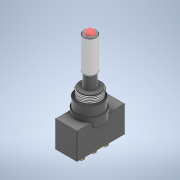
# Autodesk Inventor part: Тумблер(укороченный)
Saved by Autodesk Inventor 2020 (Build 240168000, 168)
## iProperties
Created: 2020-02-08
Part Number: Тумблер(укороченный)
Material: Типовые
Document SubType Name: Modeling
Designer: Andre
Density: 1 g/cm^3
Appearance: По умолчанию
Author: Andre
Autodesk Inventor part; units mm, degrees
ref_plane "YZ Plane" through (0, 0, 0) normal (1, 0, 0) x (0, 1, 0)
ref_plane "XZ Plane" through (0, 0, 0) normal (0, 1, 0) x (-1, 0, 0)
ref_plane "XY Plane" through (0, 0, 0) normal (0, 0, 1) x (1, 0, 0)
sketch "Эскиз1" plane through (0, 0, 0) normal (0, 1, 0) x (-1, 0, 0)
  line L0 (6, -13.1) -> (-6, -13.1)
  line L1 (-6, -13.1) -> (-6, 13.1)
  line L2 (-6, 13.1) -> (6, 13.1)
  line L3 (6, 13.1) -> (6, -13.1)
  point P0 (0, 0)
  point P1 (0, 0)
  point P2 (0, 0)
  point P3 (0, 0)
  point P4 (-5.9706, -15.2069)
  dimension "d0" = 12
  dimension "d1" = 26.2
  constraints: 8 end point, 3 coincident, 2 parallel, 1 horizontal, 1 perpendicular
  measures "d0" distance of L1.end L2.end
  measures "d1" distance of L0.end L1.end
extrude "Корпус" add sketch "Эскиз1" along normal blind 14.5
sketch "Эскиз2" plane through (0, 0, 0) normal (0, -1, 0) x (1, 0, 0)
  line L0 (3.2, 0.4) -> (-3.2, 0.4)
  line L1 (-3.2, 0.4) -> (-3.2, -0.4)
  line L2 (-3.2, -0.4) -> (3.2, -0.4)
  line L3 (3.2, -0.4) -> (3.2, 0.4)
  line L4 (3.2, -6.1) -> (-3.2, -6.1)
  line L5 (-3.2, -6.1) -> (-3.2, -6.9)
  line L6 (-3.2, -6.9) -> (3.2, -6.9)
  line L7 (3.2, -6.9) -> (3.2, -6.1)
  line L8 (-3.2, -6.9) -> (-3.2, -6.5)
  line L9 (3.2, 6.9) -> (-3.2, 6.9)
  line L10 (-3.2, 6.9) -> (-3.2, 6.1)
  line L11 (-3.2, 6.1) -> (3.2, 6.1)
  line L12 (3.2, 6.1) -> (3.2, 6.9)
  point P0 (0, 0)
  dimension "d8" = 6.4
  dimension "d9" = 0.8
  dimension "d15" = 6.4
  dimension "d16" = 0.8
  dimension "d20" = 6.4
  dimension "d21" = 0.8
  constraints: 26 end point, 6 parallel, 3 horizontal, 3 perpendicular, 1 midpoint
  measures "d8" distance of L2.end L1.end
  measures "d9" distance of L1.end L0.end
  measures "d15" distance of L6.end L5.end
  measures "d16" distance of L5.end L4.end
  measures "d20" distance of L12.start L10.end
  measures "d21" distance of L10.end L10.start
extrude "Клемы" add sketch "Эскиз2" along normal blind 4.5
chamfer "Фаска1" distance 1 angle 45 6 edges at (-3.2, -4.5, 6.5) (-3.2, -4.5, 0) (-3.2, -4.5, -6.5) (3.2, -4.5, -6.5) (3.2, -4.5, 0) (3.2, -4.5, 6.5)
sketch "Эскиз3" plane through (3.2, 0, -6.9) normal (0, 0, -1) x (-1, 0, 0)
  circle A0 centre (3.2, -7) radius 1
  point P0 (3.2, 0)
  point P1 (5.4, -4.5)
  dimension "d30" = 2
  constraints: 1 centre point
  measures "d30" diameter of A0
hole "Отверстие1" at (0, -7, -6.9) direction (0, 0, 1) diameter 2 end through all
sketch "Эскиз4" plane through (0, 14.5, 0) normal (0, 1, 0) x (1, 0, 0)
  circle A0 centre (0, 0) radius 6
  circle A1 centre (0, 0) radius 7.5
  dimension "d40" = 12
  dimension "d42" = 15
  constraints: 2 centre point, 2 coincident
  measures "d40" diameter of A0
  measures "d42" diameter of A1
extrude "Выдавливание3" add sketch "Эскиз4" along normal blind 11 contours A0
sketch "Эскиз5" plane through (0, 14.5, 0) normal (0, 1, 0) x (1, 0, 0)
  line L0 (2.2, -0.4) -> (-2.2, -0.4) projected
  circle A0 centre (0, -0.4) radius 7.5
  point P0 (0, 0)
  dimension "d45" = 15
  constraints: 1 centre point, 1 midpoint
  measures "d45" diameter of A0
extrude "Выдавливание4" add sketch "Эскиз5" along normal mid plane 5
sketch "Эскиз6" plane through (0, 17, 0.4) normal (0, 1, 0) x (1, 0, 0)
  line L0 (2.2, 0) -> (-2.2, 0) projected
  circle A0 centre (0, 0) radius 7
  point P0 (0, 0.4)
  dimension "d48" = 14
  constraints: 1 centre point, 1 midpoint
  measures "d48" diameter of A0
extrude "Выдавливание5" add sketch "Эскиз6" along normal blind 5
thread "Резьба1" size "M12x0.75" class "6g" standard "ANSI Metric M Profile" full length
fillet "Сопряжение1" radius 0.2 1 edges at (-6, 25.5, 0)
sketch "Эскиз9" plane through (0, 25.5, 0) normal (0, 1, 0) x (1, 0, 0)
  circle A0 centre (0, 0) radius 5.5
  dimension "d71" = 11
  constraints: 1 centre point, 1 coincident
  measures "d71" diameter of A0
extrude "Выдавливание6" add sketch "Эскиз9" along normal blind 0.5
sketch "Эскиз10" plane through (0, 26, 0) normal (0, 1, 0) x (1, 0, 0)
  circle A0 centre (0, 0) radius 3
  dimension "d74" = 6
  constraints: 1 centre point, 1 coincident
  measures "d74" diameter of A0
extrude "Выдавливание7" add sketch "Эскиз10" along normal blind 7
sketch "Эскиз11" plane through (0, 33, 0) normal (0, 1, 0) x (1, 0, 0)
  circle A0 centre (0, 0) radius 3.5
  dimension "d77" = 7
  constraints: 1 centre point, 1 coincident
  measures "d77" diameter of A0
extrude "Выдавливание8" add sketch "Эскиз11" along normal blind 18
fillet "Сопряжение2" radius 1 1 edges at (-3.5, 33, 0)
sketch "Эскиз12" plane through (0, 51, 0) normal (0, 1, 0) x (1, 0, 0)
  circle A0 centre (0, 0) radius 3.25
  dimension "d81" = 6.5
  constraints: 1 centre point, 1 coincident
  measures "d81" diameter of A0
extrude "Выдавливание9" add sketch "Эскиз12" along normal blind 0.5
fillet "Сопряжение3" radius 0.2 1 edges at (-3.25, 51.5, 0)
sketch "Эскиз13" plane through (0, 51.5, 0) normal (0, 1, 0) x (1, 0, 0)
  circle A0 centre (0, 0) radius 2.5
  dimension "d85" = 5
  constraints: 1 centre point, 1 coincident
  measures "d85" diameter of A0
extrude "Выдавливание10" add sketch "Эскиз13" along normal blind 2
fillet "Сопряжение4" radius 2.5 1 edges at (-2.5, 53.5, 0)
fillet "Сопряжение5" radius 0.2 1 edges at (0, 14.5, -13.1)
fillet "Сопряжение6" radius 0.2 1 edges at (0, 14.5, 13.1)
fillet "Сопряжение7" radius 0.2 6 edges at (-6, 14.4414, -13.0414) (-6, 7.15, -13.1) (-6, 14.5, -8.5) (-6, 14.4414, 13.0414) (-6, 7.15, 13.1) (-6, 14.5, 8.9)
fillet "Сопряжение8" radius 0.2 6 edges at (6, 14.4414, 13.0414) (6, 14.5, 8.9) (6, 7.15, 13.1) (6, 14.4414, -13.0414) (6, 7.15, -13.1) (6, 14.5, -8.5)
fillet "Сопряжение9" radius 0.2 8 edges at (-5.9414, 0, -13.0414) (-6, 0, 0) (-5.9414, 0, 13.0414) (0, 0, 13.1) (5.9414, 0, 13.0414) (6, 0, 0) (5.9414, 0, -13.0414) (0, 0, -13.1)
thread "Резьба2" size "M12x0.75" class "6g" standard "ANSI Metric M Profile" full length
sketch "Эскиз14" plane through (6, 12, 4.9) normal (1, 0, 0) x (0, 0, -1)
  point P0 (4.9, -12)
sketch "Эскиз15" plane through (-6, 12, -4.1) normal (-1, 0, 0) x (0, 0, 1)
  point P0 (4.1, -12)
sketch "Эскиз17" plane through (0, 25.5, 0) normal (1, 0, 0) x (0, 0, 1)
  line L0 (6, 0) -> (6, 3.5)
  line L1 (6, 3.5) -> (5.4439, 3.5)
  line L2 (5.4439, 3.5) -> (5.4439, 0)
  line L3 (5.4439, 0) -> (6, 0)
  line L4 (0, -40.6) -> (0, 47.6) projected
  constraints: 8 end point
revolve "Вращение1" cut sketch "Эскиз17" angle 360 about axis through (0, 25.5, 0) along (0, -1, 0)
sketch "Эскиз18" plane through (0, 25.5, 0) normal (1, 0, 0) x (0, 0, 1)
  line L0 (6, 0) -> (6, 3.5)
  line L1 (6, 3.5) -> (5.4439, 3.5)
  line L2 (5.4439, 3.5) -> (5.4439, 0)
  line L3 (5.4439, 0) -> (6, 0)
  line L4 (0, -40.6) -> (0, 47.6) projected
  constraints: 8 end point
revolve "Вращение2" add sketch "Эскиз18" angle 360 about axis through (0, 25.5, 0) along (0, -1, 0) separate body
sketch "Эскиз16" plane through (0, 25.5, 0) normal (-1, 0, 0) x (0, -1, 0)
  line L0 (-0.4376, -5.482) -> (-0.3751, -5.482) construction
  line L1 (0.0624, -5.9622) -> (-0.0001, -6.0823) construction
  line L2 (-0.7501, -6.0823) -> (-0.8126, -5.9622) construction
  line L3 (-0.3126, -5.482) -> (-0.3751, -5.3619) construction
  line L4 (-0.3751, -5.3619) -> (-0.4376, -5.482) construction
  line L5 (-0.7501, -6.0823) -> (-0.6876, -5.9622) construction
  line L6 (-0.3126, -5.482) -> (-0.0626, -5.9622)
  line L7 (-0.8126, -5.9622) -> (-0.6876, -5.9622) construction
  arc A0 (-0.8126, -5.9622) -> (-0.7501, -6.0002) centre (-0.7501, -5.9297) ccw construction
  line L8 (0.0624, -5.9622) -> (-0.0626, -5.9622) construction
  line L9 (-0.7501, -6.0823) -> (-0.7501, -5.9622) construction
  line L10 (-0.0001, -6.0823) -> (-0.0001, -5.9622) construction
  line L11 (-0.3751, -5.3619) -> (-0.3751, -5.4441) construction
  line L12 (-0.7501, -6.0002) -> (-0.0001, -6.0002)
  arc A1 (-0.7501, -6.0002) -> (-0.6876, -5.9622) centre (-0.7501, -5.9297) ccw
  line L13 (-0.0626, -5.9622) -> (-0.0001, -6.0823) construction
  line L14 (-0.6876, -5.9622) -> (-0.4376, -5.482)
  line L15 (-0.0001, -0.0002) -> (-0.0001, 0.0177)
  line L16 (-0.0001, 0.0177) -> (-0.0001, -0.0002)
  line L17 (-0.0001, -0.0002) -> (0.0334, -0.0002)
  arc A2 (-0.0626, -5.9622) -> (-0.0001, -6.0002) centre (-0.0001, -5.9297) ccw
  arc A3 (-0.0001, -6.0002) -> (0.0624, -5.9622) centre (-0.0001, -5.9297) ccw construction
  arc A4 (-0.3751, -5.4441) -> (-0.4376, -5.482) centre (-0.3751, -5.5145) ccw
  arc A5 (-0.3126, -5.482) -> (-0.3751, -5.4441) centre (-0.3751, -5.5145) ccw
  line L18 (-0.3751, -5.4441) -> (-0.3751, -5.482) construction
  line L19 (-0.3751, -5.482) -> (-0.3126, -5.482) construction
  dimension "d96" = 55
  dimension "d97" = 0.1201
  dimension "d98" = 0.1201
  dimension "Эскиз16_ThreadOffset" = 0
  dimension "Эскиз16_MajorRadius" = 6
  dimension "d101" = 0.75
  dimension "Эскиз16_MinorRadius" = 5.4439
  constraints: 40 end point, 12 point on circle, 10 parallel, 8 tangent, 6 centre point, 6 collinear, 2 midpoint, 2 point on line, 1 horizontal, 1 perpendicular, 3 other
  measures "d96" angle of L6 L14
  measures "d97" distance of L3.end L0.end
  measures "d98" distance of L1.end L10.end
  measures "Эскиз16_ThreadOffset" distance between parallel lines of L15 L10
  measures "Эскиз16_MajorRadius" distance from line of L12 L15.start
  measures "d101" distance from line of L1.end L9
  measures "Эскиз16_MinorRadius" distance edge to line of A5 L17
coil "Пружина1" sketch "Эскиз16" operation cut axis through (0, 25.5, 0) along (0, -1, 0) pitch 0.7508 turns 6.660007 hand right bodies 2
equation "\"d96\" = d103"
equation "\"d97\" = 0.160083 * Эскиз16_Pitch"
equation "\"d98\" = 0.160083 * Эскиз16_Pitch"
equation "\"d101\" = Эскиз16_Pitch"
equation "\"d103\" = 55deg"
equation "\"Эскиз16_Pitch\" = 0.75"
